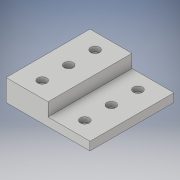
# Autodesk Inventor part: screwbaserecesed
Saved by Autodesk Inventor 2019 (Build 230136000, 136)
## iProperties
Created: 2018-12-19
Part Number: screwbaserecesed
Material: Generic
Document SubType Name: Modeling
Designer: assman
Density: 1 g/cm^3
Appearance: Default
Author: assman
Autodesk Inventor part; units mm, degrees
ref_plane "YZ Plane" through (0, 0, 0) normal (1, 0, 0) x (0, 1, 0)
ref_plane "XZ Plane" through (0, 0, 0) normal (0, 1, 0) x (-1, 0, 0)
ref_plane "XY Plane" through (0, 0, 0) normal (0, 0, 1) x (1, 0, 0)
sketch "Sketch1" plane through (0, 0, 0) normal (0, 1, 0) x (-1, 0, 0)
  line L0 (25, 25) -> (-25, 25)
  line L1 (-25, 25) -> (-25, -25)
  line L2 (-25, -25) -> (25, -25)
  line L3 (25, -25) -> (25, 25)
  line L4 (35, 0) -> (-35, 0) projected
  line L5 (0, -35) -> (0, 35) projected
  point P0 (0, 0)
  dimension "d0" = 50
  dimension "d1" = 50
  constraints: 8 end point, 2 parallel, 1 horizontal, 1 perpendicular, 2 other
  measures "d0" distance of L2.end L1.end
  measures "d1" distance of L1.end L0.end
extrude "Extrusion1" add sketch "Sketch1" along normal blind 12.85
sketch "Sketch2" plane through (0, 12.85, 0) normal (0, 1, 0) x (1, 0, 0)
  line L0 (-25, -25) -> (25, -25) projected
  line L1 (25, -25) -> (25, 25) projected
  line L2 (0, -25) -> (25, -25)
  line L3 (25, -25) -> (25, 25)
  line L4 (25, 25) -> (0, 25)
  line L5 (0, 25) -> (0, -25)
  point P0 (0, 0)
  constraints: 8 end point, 2 parallel, 1 horizontal, 1 midpoint, 1 perpendicular
extrude "Extrusion2" cut sketch "Sketch2" against normal blind 7.85
sketch "Sketch3" plane through (0, 12.85, 0) normal (0, 1, 0) x (1, 0, 0)
  line L0 (-25, -25) -> (25, -25) construction
  line L1 (-12.7037, -25) -> (-12.7037, 25.0391) construction
  line L2 (12.6423, -25) -> (12.6423, 25.0391) construction
  line L3 (-35, 0) -> (35, 0) projected
  point P0 (0, 0)
  point P1 (-12.7037, -15.7722)
  point P2 (-12.7037, 0.0196)
  point P3 (-12.7037, 15.7722)
  point P4 (12.6423, -15.7722)
  point P5 (12.6423, 0.0196)
  point P6 (12.6423, 15.7722)
  constraints: 6 point on line, 4 end point, 2 midpoint, 2 symmetric about line, 1 perpendicular, 1 vertical
hole "Hole1" at (-12.7037, 12.85, 15.7722) at (-12.7037, 12.85, -0.0196) at (-12.7037, 12.85, -15.7722) at (12.6423, 12.85, 15.7722) at (12.6423, 12.85, -0.0196) at (12.6423, 12.85, -15.7722) direction (0, -1, 0) diameter 2.4638 end through all counterbore diameter 5.37 counterbore depth 2.85
sketch "Sketch4" plane through (0, 5, 0) normal (0, 1, 0) x (1, 0, 0)
  point P0 (0, 0)
  point P1 (12.7037, -15.8336)
  point P2 (12.7037, 0)
  point P3 (12.7037, 15.8336)
hole "Hole2" at (12.7037, 5, 0) at (12.7037, 5, -15.8336) at (12.7037, 5, 15.8336) direction (0, -1, 0) diameter 2.4638 end through all counterbore diameter 5.37 counterbore depth 2.85
body "Solid1"
